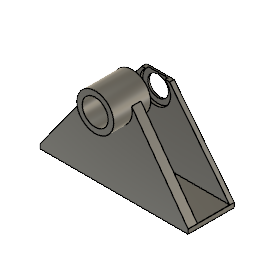
RUEDA Y ARMA v3 (Autodesk Fusion 360 design; units mm, degrees)
Autodesk Fusion 360 part; units mm, degrees
sketch "Boceto1" plane through (0, 0, 0) normal (0, 1, 0) x (1, 0, 0)
  line L0 (-49.4638, -10.4199) -> (-49.4638, -5.4199)
  line L1 (-49.4638, -5.4199) -> (110.5362, -5.4199)
  line L2 (110.5362, -5.4199) -> (110.5362, -10.4199)
  line L3 (110.5362, -10.4199) -> (45.5362, -92.882)
  line L4 (45.5362, -92.882) -> (15.5362, -92.882)
  line L5 (15.5362, -92.882) -> (-49.4638, -10.4199)
  dimension "d1" = 5
  dimension "d2" = 160
  dimension "d3" = 5
  dimension "d4" = 105
  dimension "d5" = 30
  dimension "d6" = 105
  constraint vertical L0
  constraint perpendicular L0 L1
  constraint perpendicular L1 L2
  constraint parallel L1 L4
  measures "d1" distance of L0.start L0.end
  measures "d2" distance of L0.end L1.end
  measures "d3" distance of L1.end L2.end
  measures "d4" distance of L2.end L3.end
  measures "d5" distance of L3.end L4.end
  measures "d6" distance of L0.start L4.end
extrude "Extruir1" add sketch "Boceto1" along normal blind 50 makes body 1
sketch "Boceto2" plane through (0, 0, 0) normal (0, 1, 0) x (1, 0, 0)
  line L0 (-49.5, -10.5) -> (110.5, -10.5)
  line L1 (110.5, -10.5) -> (45.555, -93.0053)
  line L2 (45.555, -93.0053) -> (15.555, -93.0053)
  line L3 (15.555, -93.0053) -> (-49.5, -10.5)
  dimension "d9" = 160
  dimension "d10" = 30
  constraint horizontal L0
  constraint parallel L0 L2
  measures "d9" distance of L0.start L0.end
  measures "d10" distance of L1.end L2.end
extrude "Extruir2" cut sketch "Boceto2" along normal blind 45 bodies 1
sketch "Boceto3" plane through (0, 0, 0) normal (0, 1, 0) x (1, 0, 0)
  circle A0 centre (30, -80) radius 16.5
  dimension "d13" = 33
  measures "d13" diameter of A0
extrude "Extruir3" cut sketch "Boceto3" along normal blind 48 bodies 1
sketch "Boceto4" plane through (0, 0, 0) normal (0, 1, 0) x (1, 0, 0)
  circle A0 centre (30, -80) radius 11
  dimension "d16" = 22
  measures "d16" diameter of A0
extrude "Extruir4" cut sketch "Boceto4" along normal blind 55 bodies 1
sketch "Boceto5" plane through (0, 0, 0) normal (0, 1, 0) x (1, 0, 0)
  line L0 (-49.5804, -10.8719) -> (110.4196, -10.8719)
  line L1 (110.4196, -10.8719) -> (42.9196, -103.9781)
  line L2 (42.9196, -103.9781) -> (17.9196, -103.9781)
  line L3 (17.9196, -103.9781) -> (-49.5804, -10.8719)
  dimension "d19" = 160
  dimension "d20" = 115
  dimension "d21" = 115
  dimension "d22" = 25
  constraint horizontal L0
  constraint parallel L0 L2
  measures "d19" distance of L0.start L0.end
  measures "d20" distance of L0.end L1.end
  measures "d21" distance of L0.start L2.end
  measures "d22" distance of L1.end L2.end
extrude "Extruir5" add sketch "Boceto5" along normal blind 10 separate body makes body 2
move_body "Alinear1" bodies 1 to x (1, 0, 0) y (0, 1, 0) z (0, 0, 1) at (-0.1166, 0, 0.4521)
combine "Combinar2" operation add target body 1 tool bodies 2
sketch "Boceto6" plane through (0, 0, 0) normal (0, 1, 0) x (1, 0, 0)
  circle A0 through (50, -90, -20) (20, -72.6795, -20) (20, -107.3205, -20)
  dimension "d25" = 40
extrude "Extruir6" cut sketch "Boceto6" along normal blind 40 contours A0 in plane through (0, -20, 0) normal (0, 1, 0) bodies 1
sketch "Boceto7" plane through (0, 0, 0) normal (0, 1, 0) x (1, 0, 0)
  circle A0 through (50, -90, -20) (20, -72.6795, -20) (20, -107.3205, -20)
  dimension "d28" = 40
extrude "Extruir7" add sketch "Boceto7" along normal blind 40 contours A0 in plane through (0, -20, 0) normal (0, 1, 0) bodies 1
sketch "Boceto8" plane through (0, 0, 0) normal (0, 1, 0) x (1, 0, 0)
  circle A0 through (44, -90, -21) (23, -77.8756, -21) (23, -102.1244, -21)
  dimension "d31" = 28
extrude "Extruir8" cut sketch "Boceto8" along normal blind 37 contours A0 in plane through (0, -21, 0) normal (0, 1, 0) bodies 1
sketch "Boceto9" plane through (0, 0, 0) normal (0, 1, 0) x (1, 0, 0)
  circle A0 centre (30, -90) radius 5
  dimension "d34" = 10
  measures "d34" diameter of A0
extrude "Extruir9" cut sketch "Boceto9" along normal blind 25 bodies 1
hole "Agujero1" at (74.4604, 23.4345, 5.8719) direction (0, 0, 1) diameter 5 depth 10 tip angle 118 bodies 1
hole "Agujero2" at (-4.9517, 24.1281, 5.8719) direction (0, 0, 1) diameter 5 depth 10 tip angle 118 bodies 1
